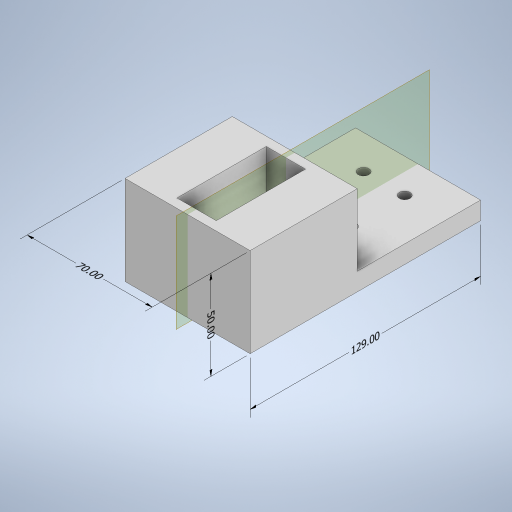
# Autodesk Inventor part: servo_piece
Saved by Autodesk Inventor 2023 (Build 270158000, 158)
## iProperties
Created: 2023-05-08
Part Number: servo_piece
Material: Genérico
Document SubType Name: Modeling
Designer: papel
Density: 1 g/cm^3
Appearance: Valor por defecto
Author: papel
Autodesk Inventor part; units mm, degrees
ref_plane "YZ Plane" through (0, 0, 0) normal (1, 0, 0) x (0, 1, 0)
ref_plane "XZ Plane" through (0, 0, 0) normal (0, 1, 0) x (-1, 0, 0)
ref_plane "XY Plane" through (0, 0, 0) normal (0, 0, 1) x (1, 0, 0)
sketch "Boceto1" plane through (0, 0, 0) normal (0, 1, 0) x (-1, 0, 0)
  line L0 (0.0239, -45) -> (35.0239, -45)
  line L1 (35.0239, -10) -> (-34.9761, -10)
  line L2 (-40.6213, -10) -> (-84.6707, -10)
  line L3 (-100, -10) -> (100, -10)
  line L4 (-100, -10) -> (100, -10)
  line L5 (105.0239, -10) -> (-104.9761, -10)
  line L6 (105.0239, -10) -> (-104.9761, -10)
  line L7 (105, 10) -> (-105, 10)
  line L8 (105, 10) -> (-105, 10)
  line L9 (0.0239, -45) -> (-34.9761, -45)
  circle A0 centre (11.5239, -60) radius 3
  circle A1 centre (11.5239, -30) radius 3
  circle A2 centre (-11.4761, -30) radius 3
  line L10 (11.5239, -30) -> (-11.4761, -60)
  line L11 (-34.9761, -79) -> (35.0239, -79)
  line L12 (-34.9761, -10) -> (-34.9761, -79)
  circle A3 centre (-11.4761, -60) radius 3
  line L13 (11.5239, -60) -> (-11.4761, -30)
  line L14 (35.0239, -45) -> (35.0239, -10)
  line L15 (35.0239, -79) -> (35.0239, -10)
  point P0 (0, 0)
  point P1 (0, 0)
  point P2 (0, 0)
  point P3 (0.0478, -10)
  point P4 (0, 0)
  point P5 (-95.8154, 10)
  dimension "d0" = 20
  dimension "d1" = 20
  dimension "d2" = 30
  dimension "d3" = 30
  dimension "d4" = 20
  dimension "d5" = 35
  dimension "d6" = 35
  dimension "d7" = 69
  constraints: 32 end point, 4 centre point, 4 point on line, 3 equal length, 3 horizontal, 2 perpendicular, 1 midpoint
  measures "d0" distance from line of L5 A1.centre
  measures "d1" distance from line of A2.centre L5
  measures "d2" distance between centres of A3 A2
  measures "d3" distance of A0.centre A1.centre
  measures "d4" distance between parallel lines of L8 L5
  measures "d5" distance of L0.start L9.end
  measures "d6" distance of L0.start L0.end
  measures "d7" distance of L12.end L1.end
extrude "Extrusión1" add sketch "Boceto1" along normal blind 10
sketch "Boceto2" plane through (0, 0, 0) normal (0, -1, 0) x (1, 0, 0)
  line L0 (-35.0239, -10) -> (34.9761, -10) projected
  line L1 (-35.0239, -10) -> (-35.0239, 50)
  line L2 (-35.0239, 50) -> (34.9761, 50)
  line L3 (34.9761, 50) -> (34.9761, -10)
  point P0 (0, 0)
  dimension "d10" = 60
  constraints: 6 end point, 2 perpendicular, 1 vertical
  measures "d10" distance of L0.start L1.end
extrude "Extrusión2" add sketch "Boceto2" against normal blind 50
sketch "Boceto3" plane through (0, 50, 0) normal (0, 1, 0) x (1, 0, 0)
  line L0 (-35.0239, 79) -> (-35.0239, -50) projected
  line L1 (-35.0239, 9.9865) -> (-35.0239, -50)
  line L2 (-11, -45.0068) -> (11, -45.0068)
  line L3 (11, -45.0068) -> (11, 4.9932)
  line L4 (11, 4.9932) -> (-11, 4.9932)
  line L5 (-11, 4.9932) -> (-11, -45.0068)
  line L6 (-11, -45.0068) -> (11, 4.9932) construction
  line L7 (11, -45.0068) -> (-11, 4.9932) construction
  point P0 (0, 0)
  point P1 (0, -20.0068)
  dimension "d13" = 22
  dimension "d14" = 50
  constraints: 14 end point, 2 midpoint, 2 parallel, 1 collinear, 1 horizontal, 1 perpendicular, 1 point on line
  measures "d13" distance of L4.end L3.end
  measures "d14" distance of L3.end L2.end
extrude "Extrusión3" cut sketch "Boceto3" against normal blind 43
ref_plane "Plano de trabajo1" through (-0.0239, 0, -79) normal (-1, 0, 0) x (0, 0, 1)
sketch "Boceto4" plane through (-0.0239, 0, -79) normal (-1, 0, 0) x (0, 0, 1)
  line L0 (69, 10) -> (0, 10) projected
  line L1 (69, 10) -> (40.4098, 10)
  line L2 (69, 10) -> (69, 50) projected
  line L3 (69, 10) -> (69, 42.6104)
  line L4 (69, 35.4459) -> (55.8036, 8.5042)
  point P0 (79, 0)
  point P1 (56.5363, 10)
  dimension "d17" = 30
  constraints: 6 end point, 3 point on line
  measures "d17" distance of L4.start L4.end
extrude "Extrusión4" add sketch "Boceto4" along normal mid plane 15
